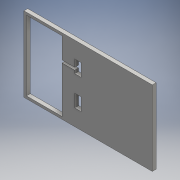
# Autodesk Inventor part: Lag 3
Saved by Autodesk Inventor 2016 (Build 200138000, 138)
## iProperties
Created: 2016-12-11
Part Number: Lag 3
Material: Generic
Document SubType Name: Modeling
Designer: Simon
Density: 1 g/cm^3
Appearance: Default
Author: Simon
Autodesk Inventor part; units mm, degrees
ref_plane "YZ Plane" through (0, 0, 0) normal (1, 0, 0) x (0, 1, 0)
ref_plane "XZ Plane" through (0, 0, 0) normal (0, 1, 0) x (-1, 0, 0)
ref_plane "XY Plane" through (0, 0, 0) normal (0, 0, 1) x (1, 0, 0)
sketch "Sketch1" plane through (0, 0, 0) normal (0, 1, 0) x (-1, 0, 0)
  line L0 (-50.5, 29.5) -> (50.5, 29.5)
  line L1 (50.5, 29.5) -> (50.5, -29.5)
  line L2 (50.5, -29.5) -> (-50.5, -29.5)
  line L3 (-50.5, -29.5) -> (-50.5, 29.5)
  line L4 (-50.5, 29.5) -> (50.5, -29.5) construction
  line L5 (50.5, 29.5) -> (-50.5, -29.5) construction
  line L6 (5.5, 16.6667) -> (10.5, 16.6667)
  line L7 (10.5, 6.6667) -> (5.5, 6.6667)
  line L8 (5.5, 6.6667) -> (5.5, 16.6667)
  line L9 (5.5, 16.6667) -> (10.5, 6.6667) construction
  line L10 (10.5, 16.6667) -> (5.5, 6.6667) construction
  line L11 (5.5, -6.6667) -> (10.5, -6.6667)
  line L12 (10.5, -16.6667) -> (5.5, -16.6667)
  line L13 (5.5, -16.6667) -> (5.5, -6.6667)
  line L14 (5.5, -6.6667) -> (10.5, -16.6667) construction
  line L15 (10.5, -6.6667) -> (5.5, -16.6667) construction
  line L16 (10.5, 10) -> (20.5, 10)
  line L17 (20.5, 11) -> (20.5, 9)
  line L18 (20.5, 9) -> (10.5, 9)
  line L19 (20.5, 11) -> (10.5, 11)
  line L20 (48.5, 27.5) -> (20.5, 27.5)
  line L21 (20.5, 27.5) -> (20.5, -27.5)
  line L22 (20.5, -27.5) -> (48.5, -27.5)
  line L23 (48.5, -27.5) -> (48.5, 27.5)
  line L24 (10.5, 16.6667) -> (10.5, 13.3333)
  line L25 (10.5, 13.3333) -> (10.5, 10)
  line L26 (10.5, 10) -> (10.5, 6.6667)
  line L27 (10.5, -16.6667) -> (10.5, -13.3333)
  line L28 (10.5, -13.3333) -> (10.5, -10)
  line L29 (10.5, -10) -> (10.5, -6.6667)
  line L30 (8, -11.6667) -> (8, 11.6667)
  line L31 (-50.5, 0) -> (50.5, 0)
  point P0 (0, 0)
  point P1 (0, 29.5)
  point P2 (0, -29.5)
  point P3 (0, 0)
  point P4 (8, 0)
  dimension "d0" = 101
  dimension "d1" = 59
  dimension "d7" = 5
  dimension "d8" = 10
  dimension "d9" = 5
  dimension "d10" = 10
  dimension "d11" = 10
  dimension "d12" = 2
  dimension "d16" = 2
  dimension "d17" = 2
  dimension "d18" = 2
  dimension "d19" = 28
  dimension "d20" = 20
  constraints: 64 end point, 11 midpoint, 7 equal length, 6 horizontal, 6 point on line, 5 collinear, 4 perpendicular, 4 vertical
  measures "d0" distance of L1.end L2.end
  measures "d1" distance of L0.end L1.end
  measures "d7" distance of L7.start L7.end
  measures "d8" distance of L7.start L6.end
  measures "d9" distance of L12.start L12.end
  measures "d10" distance of L11.end L12.start
  measures "d11" distance of L16.start L16.end
  measures "d12" distance between parallel lines of L18 L19
  measures "d16" distance between parallel lines of L1 L23
  measures "d17" distance between parallel lines of L2 L22
  measures "d18" distance between parallel lines of L0 L20
  measures "d19" distance of L21.end L22.end
  measures "d20" distance from line of L16 L28.end
extrude "Extrusion2" add sketch "Sketch1" along normal blind 3 contours L0 L1 L31 L23 L20 L21 L19 L25 L24 L6 L8 L7 L30 L3 | L31 L21 L22 L23 L1 L2 L3 | L30 L7 L26 L18 L21 L31
body "Solid2"
